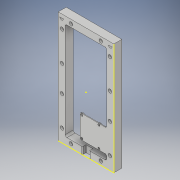
# Autodesk Inventor part: led_matrix_frame
Saved by Autodesk Inventor 2019 (Build 230136000, 136)
## iProperties
Created: 2019-01-11
Part Number: led_matrix_frame
Material: Generic
Document SubType Name: Modeling
Designer: Alex
Density: 1 g/cm^3
Appearance: Default
Author: Alex
Autodesk Inventor part; units mm, degrees
ref_plane "YZ Plane" through (0, 0, 0) normal (1, 0, 0) x (0, 1, 0)
ref_plane "XZ Plane" through (0, 0, 0) normal (0, 1, 0) x (-1, 0, 0)
ref_plane "XY Plane" through (0, 0, 0) normal (0, 0, 1) x (1, 0, 0)
sketch "Sketch1" plane through (0, 0, 0) normal (0, 0, 1) x (1, 0, 0)
  line L0 (-79.5, -159.5) -> (79.5, -159.5)
  line L1 (79.5, -159.5) -> (79.5, 159.5)
  line L2 (79.5, 159.5) -> (-79.5, 159.5)
  line L3 (-79.5, 159.5) -> (-79.5, -159.5)
  line L4 (-79.5, -159.5) -> (79.5, 159.5) construction
  line L5 (79.5, -159.5) -> (-79.5, 159.5) construction
  line L6 (-59.5, -139.5) -> (59.5, -139.5)
  line L7 (59.5, -139.5) -> (59.5, 139.5)
  line L8 (59.5, 139.5) -> (-59.5, 139.5)
  line L9 (-59.5, 139.5) -> (-59.5, -139.5)
  line L10 (-59.5, -139.5) -> (59.5, 139.5) construction
  line L11 (59.5, -139.5) -> (-59.5, 139.5) construction
  circle A0 centre (68.5, -122.5) radius 1
  circle A1 centre (42.5, -148.5) radius 1
  circle A2 centre (68.5, -37.5) radius 1
  circle A3 centre (-68.5, -37.5) radius 1
  circle A4 centre (-68.5, -122.5) radius 1
  circle A5 centre (-42.5, -148.5) radius 1
  circle A6 centre (68.5, 122.5) radius 1
  circle A7 centre (42.5, 148.5) radius 1
  circle A8 centre (68.5, 37.5) radius 1
  circle A9 centre (-68.5, 37.5) radius 1
  circle A10 centre (-68.5, 122.5) radius 1
  circle A11 centre (-42.5, 148.5) radius 1
  circle A12 centre (-42.5, 148.5) radius 2
  circle A13 centre (-68.5, 122.5) radius 2
  circle A14 centre (42.5, 148.5) radius 2
  circle A15 centre (68.5, 122.5) radius 2
  circle A16 centre (68.5, 37.5) radius 2
  circle A17 centre (-68.5, 37.5) radius 2
  circle A18 centre (-68.5, -37.5) radius 2
  circle A19 centre (-68.5, -122.5) radius 2
  circle A20 centre (-42.5, -148.5) radius 2
  circle A21 centre (42.5, -148.5) radius 2
  circle A22 centre (68.5, -122.5) radius 2
  circle A23 centre (68.5, -37.5) radius 2
  point P0 (0, 0)
  dimension "d0" = 159
  dimension "d1" = 319
  dimension "d2" = 119
  dimension "d3" = 279
  dimension "d4" = 2
  dimension "d5" = 11
  dimension "d6" = 37
  dimension "d7" = 2
  dimension "d8" = 11
  dimension "d9" = 37
  dimension "d10" = 2
  dimension "d11" = 11
  dimension "d12" = 122
  dimension "d13" = 4
  dimension "d14" = 4
  dimension "d15" = 4
  dimension "d16" = 4
  dimension "d17" = 4
  dimension "d18" = 4
  dimension "d19" = 4
  dimension "d20" = 4
  dimension "d21" = 4
  dimension "d22" = 4
  dimension "d23" = 4
  dimension "d24" = 4
  constraints: 24 centre point, 24 end point, 12 coincident, 4 midpoint, 4 parallel, 2 horizontal, 2 perpendicular
  measures "d0" distance of L2.end L1.end
  measures "d1" distance of L1.end L0.end
  measures "d2" distance of L8.end L7.end
  measures "d3" distance of L7.end L6.end
  measures "d4" diameter of A0
  measures "d5" distance from line of L1 A0.centre
  measures "d6" distance from line of L0 A0.centre
  measures "d7" diameter of A1
  measures "d8" distance from line of A1.centre L0
  measures "d9" distance from line of A1.centre L1
  measures "d10" diameter of A2
  measures "d11" distance from line of A2.centre L1
  measures "d12" distance from line of L0 A2.centre
  measures "d13" diameter of A12
  measures "d14" diameter of A13
  measures "d15" diameter of A14
  measures "d16" diameter of A15
  measures "d17" diameter of A16
  measures "d18" diameter of A17
  measures "d19" diameter of A18
  measures "d20" diameter of A19
  measures "d21" diameter of A20
  measures "d22" diameter of A21
  measures "d23" diameter of A22
  measures "d24" diameter of A23
extrude "Extrusion1" add sketch "Sketch1" along normal blind 23 contours L3 L2 L1 L0
sketch "Sketch2" plane through (0, 0, 23) normal (0, 0, 1) x (1, 0, 0)
  circle A0 centre (42.5, -148.5) radius 2 projected
  circle A1 centre (42.5, -148.5) radius 5
  circle A2 centre (68.5, -122.5) radius 2 projected
  circle A3 centre (68.5, -122.5) radius 5
  circle A4 centre (68.5, -37.5) radius 2 projected
  circle A5 centre (68.5, -37.5) radius 5
  circle A6 centre (-42.5, -148.5) radius 5
  circle A7 centre (-68.5, -122.5) radius 5
  circle A8 centre (-68.5, -37.5) radius 5
  circle A9 centre (-68.5, 37.5) radius 5
  circle A10 centre (-68.5, 122.5) radius 5
  circle A11 centre (-42.5, 148.5) radius 5
  circle A12 centre (42.5, 148.5) radius 5
  circle A13 centre (68.5, 122.5) radius 5
  circle A14 centre (68.5, 37.5) radius 5
  point P0 (0, 0)
  dimension "d27" = 10
  dimension "d28" = 10
  dimension "d29" = 10
  constraints: 12 centre point, 3 coincident
  measures "d27" diameter of A1
  measures "d28" diameter of A3
  measures "d29" diameter of A5
extrude "Extrusion2" cut sketch "Sketch2" against normal blind 5
sketch "Sketch3" plane through (0, 0, 23) normal (0, 0, 1) x (1, 0, 0)
  circle A0 centre (-69.5, 149.5) radius 5
  line L0 (79.5, 159.5) -> (-79.5, 159.5) projected
  line L1 (-79.5, 159.5) -> (-79.5, -159.5) projected
  line L2 (0, 115.3552) -> (0, 76.8376)
  circle A1 centre (69.5, 149.5) radius 5
  point P0 (0, 0)
  dimension "d32" = 10
  dimension "d33" = 10
  dimension "d34" = 10
  constraints: 2 centre point, 2 end point, 1 symmetric about line, 1 vertical, 1 other
  measures "d32" diameter of A0
  measures "d33" distance from line of L0 A0.centre
  measures "d34" distance from line of L1 A0.centre
extrude "Extrusion3" cut sketch "Sketch3" against normal blind 11.5
sketch "Sketch4" plane through (0, 0, 23) normal (0, 0, 1) x (1, 0, 0)
  circle A0 centre (-69.5, 149.5) radius 5 projected
  line L0 (-74.5, 149.5) -> (-64.5, 149.5)
  circle A1 centre (69.5, 149.5) radius 5 projected
  line L1 (64.5, 149.5) -> (74.5, 149.5)
  point P0 (0, 0)
  constraints: 4 end point, 4 point on circle, 2 horizontal
extrude "Extrusion4" add sketch "Sketch4" against normal blind 5.75 contours L0 A0 | L1 A1 picked at (-70.091, 152.6074) picked at (68.909, 152.6074)
sketch "Sketch5" plane through (0, 0, 0) normal (0, 0, -1) x (-1, 0, 0)
  circle A0 centre (-55.5, -152) radius 1.5
  line L0 (79.5, -159.5) -> (-79.5, -159.5) projected
  line L1 (-79.5, -159.5) -> (-79.5, 159.5) projected
  circle A1 centre (55.5, 152) radius 1.5
  line L2 (-79.5, 159.5) -> (79.5, 159.5) projected
  line L3 (79.5, 159.5) -> (79.5, -159.5) projected
  point P0 (0, 0)
  dimension "d39" = 3
  dimension "d40" = 7.5
  dimension "d41" = 24
  dimension "d42" = 3
  dimension "d43" = 7.5
  dimension "d44" = 24
  constraints: 2 centre point
  measures "d39" diameter of A0
  measures "d40" distance from line of L0 A0.centre
  measures "d41" distance from line of A0.centre L1
  measures "d42" diameter of A1
  measures "d43" distance from line of L2 A1.centre
  measures "d44" distance from line of L3 A1.centre
extrude "Extrusion5" cut sketch "Sketch5" against normal blind 5 contours A0 | A1
sketch "Sketch6" plane through (0, 0, 23) normal (0, 0, 1) x (1, 0, 0)
  line L0 (-79.5, -159.5) -> (79.5, -159.5) projected
  line L1 (79.5, -159.5) -> (79.5, 159.5) projected
  point P0 (0, 0)
sketch "Sketch7" plane through (0, 0, 23) normal (0, 0, 1) x (1, 0, 0)
  point P0 (0, 0)
sketch "Sketch8" plane through (0, 0, 23) normal (0, 0, 1) x (1, 0, 0)
  line L0 (-16.5, -124.5) -> (-16.5, -58.5)
  line L1 (-79.5, -159.5) -> (79.5, -159.5) projected
  line L2 (79.5, -159.5) -> (79.5, 159.5) projected
  line L3 (59.5, -139.5) -> (59.5, 139.5) projected
  line L4 (-16.5, -58.5) -> (59.5, -58.5)
  line L5 (-16.5, -124.5) -> (59.5, -124.5)
  line L6 (59.5, 139.5) -> (59.5, -139.5) projected
  point P0 (0, 0)
  constraints: 6 end point, 2 point on line, 1 parallel, 1 perpendicular
sketch "Sketch9" plane through (0, 0, 23) normal (0, 0, 1) x (1, 0, 0)
  point P0 (0, 0)
sketch "Sketch10" plane through (0, 0, 23) normal (0, 0, 1) x (1, 0, 0)
  point P0 (0, 0)
sketch "Sketch11" plane through (0, 0, 23) normal (0, 0, 1) x (1, 0, 0)
  point P0 (0, 0)
sketch "Sketch12" plane through (0, 0, 23) normal (0, 0, 1) x (1, 0, 0)
  point P0 (0, 0)
extrude "Extrusion6" add sketch "Sketch8" against normal blind 2
fillet "Fillet1" radius 5 6 edges at (59.5, -139.5, 11.5) (59.5, -58.5, 22) (-59.5, -139.5, 11.5) (59.5, -124.5, 22) (-59.5, 139.5, 11.5) (59.5, 139.5, 11.5)
fillet "Fillet2" radius 2 2 edges at (-16.5, -58.5, 22) (-16.5, -124.5, 22)
sketch "Sketch13" plane through (0, 0, 23) normal (0, 0, 1) x (1, 0, 0)
  point P0 (0, 0)
sketch "Sketch14" plane through (0, 0, 23) normal (0, 0, 1) x (1, 0, 0)
  circle A0 centre (-11.8564, -120.5) radius 1.5
  circle A1 centre (-11.8564, -62.5) radius 1.5
  circle A2 centre (37.1436, -120.5) radius 1.5
  circle A3 centre (37.1436, -62.5) radius 1.5
  line L0 (-14.5, -124.5) -> (54.5, -124.5) projected
  point P0 (0, 0)
  dimension "d58" = 3
  dimension "d59" = 3
  dimension "d60" = 58
  dimension "d61" = 3
  dimension "d62" = 3
  dimension "d63" = 49
  dimension "d64" = 49
  dimension "d65" = 4
  constraints: 4 centre point
  measures "d58" diameter of A0
  measures "d59" diameter of A1
  measures "d60" distance of A0.centre A1.centre
  measures "d61" diameter of A2
  measures "d62" diameter of A3
  measures "d63" distance of A3.centre A1.centre
  measures "d64" distance of A2.centre A0.centre
  measures "d65" distance from line of L0 A0.centre
extrude "Extrusion7" cut sketch "Sketch14" against normal blind 20
fillet "Fillet3" radius 5 1 edges at (59.5, -91.5, 21)
sketch "Sketch15" plane through (0, 0, 21) normal (0, 0, -1) x (-1, 0, 0)
  circle A0 centre (-37.1436, -62.5) radius 1.5 projected
  circle A1 centre (-37.1436, -120.5) radius 1.5 projected
  circle A2 centre (-37.1436, -62.5) radius 1.5 projected
  circle A3 centre (-37.1436, -62.5) radius 4
  circle A4 centre (11.8564, -62.5) radius 1.5 projected
  circle A5 centre (11.8564, -62.5) radius 4
  circle A6 centre (11.8564, -120.5) radius 1.5 projected
  circle A7 centre (11.8564, -120.5) radius 4
  circle A8 centre (-37.1436, -120.5) radius 1.5 projected
  circle A9 centre (-37.1436, -120.5) radius 4
  point P0 (0, 0)
  dimension "d71" = 8
  dimension "d72" = 8
  dimension "d73" = 8
  dimension "d74" = 8
  constraints: 4 centre point, 4 coincident
  measures "d71" diameter of A3
  measures "d72" diameter of A5
  measures "d73" diameter of A7
  measures "d74" diameter of A9
extrude "Extrusion8" add sketch "Sketch15" along normal blind 2
sketch "Sketch16" plane through (0, 0, 23) normal (0, 0, 1) x (1, 0, 0)
  circle A0 centre (-11.8564, -62.5) radius 1.5 projected
  circle A1 centre (-11.8564, -62.5) radius 3
  circle A2 centre (37.1436, -62.5) radius 1.5 projected
  circle A3 centre (37.1436, -62.5) radius 3
  circle A4 centre (37.1436, -120.5) radius 1.5 projected
  circle A5 centre (37.1436, -120.5) radius 3
  circle A6 centre (-11.8564, -120.5) radius 3
  point P0 (0, 0)
  dimension "d77" = 6
  dimension "d78" = 6
  dimension "d79" = 6
  dimension "d80" = 6
  constraints: 4 centre point, 3 coincident
  measures "d77" diameter of A1
  measures "d78" diameter of A3
  measures "d79" diameter of A5
  measures "d80" diameter of A6
extrude "Extrusion9" cut sketch "Sketch16" against normal blind 1.5
sketch "Sketch17" plane through (-79.5, -159.5, 0) normal (0, -1, 0) x (1, 0, 0)
  line L0 (69.5, 23) -> (89.5, 23)
  line L1 (89.5, 23) -> (89.5, 13)
  line L2 (89.5, 13) -> (69.5, 13)
  line L3 (69.5, 13) -> (69.5, 23)
  line L4 (0, 23) -> (159, 23) projected
  line L5 (0, 0) -> (0, 23) projected
  point P0 (79.5, 0)
  dimension "d83" = 20
  dimension "d84" = 10
  dimension "d85" = 69.5
  constraints: 8 end point, 2 parallel, 1 collinear, 1 horizontal, 1 perpendicular
  measures "d83" distance of L1.end L2.end
  measures "d84" distance of L0.end L1.end
  measures "d85" distance between parallel lines of L5 L3
extrude "Extrusion10" cut sketch "Sketch17" against normal blind 21
fillet "Fillet4" radius 2 4 edges at (-10, -149.5, 13) (-10, -149.5, 23) (10, -149.5, 23) (10, -149.5, 13)
body "Solid1"
